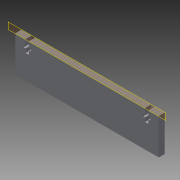
# Autodesk Inventor part: baseBoxShortSide
Saved by Autodesk Inventor 2013 (Build 170138000, 138)
## iProperties
Created: 2014-06-24
Part Number: baseBoxShortSide
Material: Generic
Document SubType Name: Modeling
Designer: Nano
Density: 1 g/cm^3
Author: Nano
Autodesk Inventor part; units mm, degrees
ref_plane "YZ Plane" through (0, 0, 0) normal (1, 0, 0) x (0, 1, 0)
ref_plane "XZ Plane" through (0, 0, 0) normal (0, 1, 0) x (-1, 0, 0)
ref_plane "XY Plane" through (0, 0, 0) normal (0, 0, 1) x (1, 0, 0)
ref_plane "Work Plane1" through (0, 0, 0) normal (0, 0, 1) x (1, 0, 0)
sketch "Sketch1" plane through (0, 0, 0) normal (0, 0, 1) x (1, 0, 0)
  line L0 (-77.8391, 0) -> (-108.8361, 0) projected
  line L1 (-108.8361, -33.02) -> (-108.8361, 0) projected
  line L2 (-77.8391, -33.02) -> (-108.8361, -33.02) projected
  line L3 (-77.8391, -33.02) -> (-77.8391, 0) projected
  line L4 (-152.4, 0) -> (0, 0) construction
  line L5 (-152.4, 0) -> (-152.4, 6.35) construction
  line L6 (0, 0) -> (0, 6.35) construction
  line L7 (-152.4, 0) -> (0, 0)
  line L8 (0, 0) -> (0, -38.1)
  line L9 (0, -38.1) -> (-152.4, -38.1)
  line L10 (-152.4, -38.1) -> (-152.4, 0)
  line L11 (-137.8458, 6.35) -> (-137.8458, 0)
  line L12 (-141.5542, 6.35) -> (-141.5542, 0)
  line L13 (-14.5542, 6.35) -> (-14.5542, 0)
  line L14 (-10.8458, 6.35) -> (-10.8458, 0)
  line L15 (-141.5542, 0) -> (-137.8458, 0)
  line L16 (-137.8458, 0) -> (-137.8458, -12.7)
  line L17 (-137.8458, -12.7) -> (-141.5542, -12.7)
  line L18 (-141.5542, -12.7) -> (-141.5542, 0)
  line L19 (-14.5542, 0) -> (-10.8458, 0)
  line L20 (-10.8458, 0) -> (-10.8458, -12.7)
  line L21 (-10.8458, -12.7) -> (-14.5542, -12.7)
  line L22 (-14.5542, -12.7) -> (-14.5542, 0)
  line L23 (-16.637, -5.7726) -> (-8.763, -5.7726)
  line L24 (-8.763, -5.7726) -> (-8.763, -8.5666)
  line L25 (-8.763, -8.5666) -> (-16.637, -8.5666)
  line L26 (-16.637, -8.5666) -> (-16.637, -5.7726)
  line L27 (-143.637, -5.7726) -> (-135.763, -5.7726)
  line L28 (-135.763, -5.7726) -> (-135.763, -8.5666)
  line L29 (-135.763, -8.5666) -> (-143.637, -8.5666)
  line L30 (-143.637, -8.5666) -> (-143.637, -5.7726)
  dimension "d0" = 38.1
  dimension "d1" = 12.7
  dimension "d2" = 7.874
  dimension "d3" = 2.794
  dimension "d6" = 2.0828
  dimension "d7" = 2.0828
  dimension "d8" = 7.874
  dimension "d9" = 2.0828
  dimension "d10" = 2.0828
  constraints: 48 end point, 10 parallel, 8 vertical, 5 horizontal, 5 perpendicular, 8 other
  measures "d0" distance of L7.end L8.end
  measures "d1" distance of L15.end L16.end
  measures "d2" distance of L24.end L25.end
  measures "d3" distance of L23.end L24.end
  measures "d6" distance between parallel lines of L26 L22
  measures "d7" distance between parallel lines of L20 L24
  measures "d8" distance of L28.end L29.end
  measures "d9" distance between parallel lines of L18 L30
  measures "d10" distance between parallel lines of L28 L16
extrude "Extrusion1" add sketch "Sketch1" against normal blind 6.35 contours L3 L2 L1 L0 | L7 L22 L23 L26 L25 L21 L20 L24 L8 L9 L10 L18 L27 L30 L29 L17 L16 L28 L1 L2 L3
equation "\"d6\" = d7"
equation "\"d9\" = d10"
body "Solid1"
